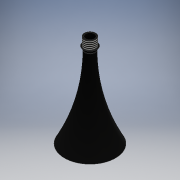
# Autodesk Inventor part: Horn_D
Saved by Autodesk Inventor 2016 (Build 200138000, 138)
## iProperties
Created: 2016-05-21
Part Number: Horn_D
Material: Steel, Cast
Document SubType Name: Modeling
Designer: agmle
Density: 7.85 g/cm^3
Appearance: Glossy - Black
Author: agmle
Autodesk Inventor part; units mm, degrees
ref_plane "YZ Plane" through (0, 0, 0) normal (1, 0, 0) x (0, 1, 0)
ref_plane "XZ Plane" through (0, 0, 0) normal (0, 1, 0) x (-1, 0, 0)
ref_plane "XY Plane" through (0, 0, 0) normal (0, 0, 1) x (1, 0, 0)
sketch "Sketch1" plane through (0, 0, 0) normal (0, 1, 0) x (-1, 0, 0)
  line L0 (0, 0) -> (10.5, 0) construction
  line L1 (0, 0) -> (0, -171.8) construction
  line L2 (0, -171.8) -> (47.15, -171.8) construction
  line L3 (0, -21.8) -> (9.5, -21.8) construction
  line L4 (0, -20.8) -> (9.5, -20.8) construction
  line L5 (0, -15.3) -> (12.6, -15.3) construction
  line L6 (8, 0) -> (10.5, 0)
  line L7 (10.5, 0) -> (10.5, -15.3)
  line L8 (10.5, -15.3) -> (12.6, -15.3)
  line L9 (12.6, -15.3) -> (9.5, -20.8)
  line L10 (9.5, -20.8) -> (9.5, -21.8)
  line L11 (8, 0) -> (8, -21.8)
  arc A0 (9.5, -21.8) -> (47.15, -171.8) centre (327.1298, -21.8) ccw
  arc A1 (8, -21.8) -> (45.4494, -171.8) centre (327.1298, -21.8) ccw
  arc A2 (45.4494, -171.8) -> (47.15, -171.8) centre (46.2997, -171.3472) ccw
  dimension "d0" = 150
  dimension "d1" = 1
  dimension "d2" = 5.5
  dimension "d3" = 15.3
  dimension "d4" = 47.15
  dimension "d5" = 9.5
  dimension "d6" = 9.5
  dimension "d7" = 12.6
  dimension "d8" = 10.5
  dimension "d9" = 1.5
  constraints: 24 end point, 7 point on line, 6 point on circle, 4 horizontal, 3 centre point, 2 collinear, 2 perpendicular, 2 tangent, 1 concentric, 1 parallel, 1 vertical
  measures "d0" distance between parallel lines of L3 L2
  measures "d1" distance between parallel lines of L4 L3
  measures "d2" distance between parallel lines of L5 L4
  measures "d3" distance between parallel lines of L0 L5
  measures "d4" distance of L1.end L2.end
  measures "d5" distance of L3.start L3.end
  measures "d6" distance of L4.start L4.end
  measures "d7" distance of L5.start L5.end
  measures "d8" distance of L0.start L0.end
  measures "d9" distance between parallel lines of L10 L11
revolve "Revolution1" add sketch "Sketch1" angle 360 about axis through (0, 0, 0) along (0, 0, -1)
thread "Thread1" size "M22x3" class "6g" standard "ANSI Metric M Profile" full length
equation "\"d0\" = Flare_Length"
equation "\"d1\" = Transition_Length"
equation "\"d2\" = Mount_Flange_Length"
equation "\"d3\" = Mount_Length"
equation "\"d4\" = Flare_Diameter"
equation "\"d6\" = Tail_Diameter"
equation "\"d7\" = Mount_Flange_Diameter"
equation "\"d8\" = Mount_Diameter"
equation "\"d9\" = Bell_Thickness"
equation "\"Transition_Length\" = 1"
equation "\"Flare_Length\" = 150"
equation "\"Mount_Flange_Length\" = 5.5"
equation "\"Mount_Length\" = 15.3"
equation "\"Flare_Diameter\" = 47.15"
equation "\"Tail_Diameter\" = 9.5"
equation "\"Mount_Flange_Diameter\" = 12.6"
equation "\"Mount_Diameter\" = 10.5"
equation "\"Bell_Thickness\" = 1.5"
body "Solid1"
